Autodesk Fusion 360 part; units mm, degrees
note: some values were not read from the file. Set by a fixed rule: which sketch regions a step uses.
(part 7 of 20)
  spline S36 degree 5 poles (-17.8091, -22.9448) (-17.8092, -22.9448) (-17.8093, -22.945) (-17.8095, -22.9453) (-17.8098, -22.9457) (-17.8103, -22.9463) (-17.8108, -22.9469) (-17.8114, -22.9477) (-17.812, -22.9486) (-17.8127, -22.9496) (-17.8135, -22.9506) (-17.8144, -22.9518) (-17.8153, -22.953) (-17.8162, -22.9543) (-17.8172, -22.9557) (-17.8183, -22.9572) (-17.8195, -22.9588) (-17.8207, -22.9604) (-17.8219, -22.9622) (-17.8232, -22.964) (-17.8246, -22.9659) (-17.826, -22.9679) (-17.8274, -22.9699) (-17.8289, -22.9721) (-17.8305, -22.9743) (-17.8321, -22.9766) (-17.8337, -22.979) (-17.8354, -22.9814) (-17.8372, -22.984) (-17.8389, -22.9866) (-17.8408, -22.9893) (-17.8427, -22.992) (-17.8446, -22.9948) (-17.8465, -22.9978) (-17.8485, -23.0007) (-17.8506, -23.0038) (-17.8527, -23.0069) (-17.8548, -23.0101) (-17.857, -23.0134) (-17.8592, -23.0167) (-17.8614, -23.0201) (-17.8637, -23.0236) (-17.866, -23.0271) (-17.8683, -23.0308) (-17.8707, -23.0344) (-17.8731, -23.0382) (-17.8756, -23.042) (-17.8781, -23.0459) (-17.8806, -23.0499) (-17.8831, -23.0539) (-17.8857, -23.058) (-17.8883, -23.0621) (-17.891, -23.0664) (-17.8937, -23.0706) (-17.8964, -23.075) (-17.8991, -23.0794) (-17.9019, -23.0839) (-17.9047, -23.0884) (-17.9075, -23.093) (-17.9103, -23.0977) (-17.9132, -23.1024) (-17.9161, -23.1072) (-17.9191, -23.1121) (-17.922, -23.117) (-17.925, -23.122) (-17.928, -23.127) (-17.931, -23.1321) (-17.9341, -23.1373) (-17.9372, -23.1425) (-17.9403, -23.1478) (-17.9434, -23.1531) (-17.9466, -23.1585) (-17.9497, -23.164) (-17.9529, -23.1695) (-17.9562, -23.1751) (-17.9594, -23.1807) (-17.9627, -23.1864) (-17.9659, -23.1921) (-17.9692, -23.1979) (-17.9726, -23.2038) (-17.9759, -23.2097) (-17.9793, -23.2157) (-17.9826, -23.2217) (-17.986, -23.2278) (-17.9895, -23.234) (-17.9929, -23.2402) (-17.9963, -23.2464) (-17.9998, -23.2527) (-18.0033, -23.2591) (-18.0068, -23.2655) (-18.0103, -23.272) (-18.0139, -23.2785) (-18.0174, -23.2851) (-18.021, -23.2918) (-18.0246, -23.2984) (-18.0282, -23.3052) (-18.0318, -23.312) (-18.0354, -23.3188) (-18.039, -23.3257) (-18.0427, -23.3327) (-18.0464, -23.3397) (-18.0501, -23.3468) (-18.0538, -23.3539) (-18.0575, -23.361) (-18.0612, -23.3683) (-18.0649, -23.3755) (-18.0687, -23.3828) (-18.0724, -23.3902) (-18.0762, -23.3976) (-18.08, -23.4051) (-18.0838, -23.4126) (-18.0876, -23.4202) (-18.0914, -23.4278) (-18.0952, -23.4355) (-18.0991, -23.4432) (-18.1029, -23.451) (-18.1068, -23.4588) (-18.1106, -23.4666) (-18.1145, -23.4746) (-18.1184, -23.4825) (-18.1223, -23.4905) (-18.1262, -23.4986) (-18.1301, -23.5067) (-18.134, -23.5149) (-18.1379, -23.5231) (-18.1419, -23.5313) (-18.1458, -23.5396) (-18.1498, -23.548) (-18.1537, -23.5564) (-18.1577, -23.5648) (-18.1617, -23.5733) (-18.1657, -23.5818) (-18.1696, -23.5904) (-18.1736, -23.5991) (-18.1776, -23.6077) (-18.1816, -23.6165) (-18.1857, -23.6252) (-18.1897, -23.634) (-18.1937, -23.6429) (-18.1977, -23.6518) (-18.2018, -23.6607) (-18.2058, -23.6697) (-18.2098, -23.6788) (-18.2139, -23.6879) (-18.2179, -23.697) (-18.222, -23.7062) (-18.226, -23.7154) (-18.2301, -23.7247) (-18.2342, -23.734) (-18.2383, -23.7433) (-18.2423, -23.7527) (-18.2464, -23.7622) (-18.2505, -23.7716) (-18.2546, -23.7812) (-18.2587, -23.7907) (-18.2627, -23.8004) (-18.2668, -23.81) (-18.2709, -23.8197) (-18.275, -23.8295) (-18.2791, -23.8393) (-18.2832, -23.8491) (-18.2873, -23.859) (-18.2914, -23.8689) (-18.2955, -23.8788) (-18.2996, -23.8888) (-18.3038, -23.8989) (-18.3079, -23.909) (-18.312, -23.9191) (-18.3161, -23.9292) (-18.3202, -23.9395) (-18.3243, -23.9497) (-18.3284, -23.96) (-18.3325, -23.9703) (-18.3366, -23.9807) (-18.3408, -23.9911) (-18.3449, -24.0016) (-18.349, -24.0121) (-18.3531, -24.0226) (-18.3572, -24.0332) (-18.3613, -24.0438) (-18.3654, -24.0545) (-18.3695, -24.0652) (-18.3736, -24.0759) (-18.3777, -24.0867) (-18.3818, -24.0975) (-18.3859, -24.1084) (-18.39, -24.1193) (-18.3941, -24.1302) (-18.3982, -24.1412) (-18.4023, -24.1522) (-18.4064, -24.1633) (-18.4105, -24.1744) (-18.4146, -24.1855) (-18.4187, -24.1967) (-18.4228, -24.2079) (-18.4269, -24.2191) (-18.4309, -24.2304) (-18.435, -24.2417) (-18.4391, -24.2531) (-18.4431, -24.2645) (-18.4472, -24.276) (-18.4513, -24.2874) (-18.4553, -24.299) (-18.4594, -24.3105) (-18.4634, -24.3221) (-18.4675, -24.3337) (-18.4715, -24.3454) (-18.4756, -24.3571) (-18.4796, -24.3689) (-18.4836, -24.3806) (-18.4877, -24.3925) (-18.4917, -24.4043) (-18.4957, -24.4162) (-18.4997, -24.4281) (-18.5037, -24.4401) (-18.5077, -24.4521) (-18.5117, -24.4642) (-18.5157, -24.4762) (-18.5197, -24.4884) (-18.5237, -24.5005) (-18.5277, -24.5127) (-18.5316, -24.5249) (-18.5356, -24.5372) (-18.5395, -24.5495) (-18.5435, -24.5618) (-18.5475, -24.5742) (-18.5514, -24.5866) (-18.5553, -24.599) (-18.5593, -24.6115) (-18.5632, -24.624) (-18.5671, -24.6365) (-18.571, -24.6491) (-18.5749, -24.6617) (-18.5788, -24.6744) (-18.5827, -24.6871) (-18.5866, -24.6998) (-18.5905, -24.7125) (-18.5943, -24.7253) (-18.5982, -24.7382) (-18.6021, -24.751) (-18.6059, -24.7639) (-18.609, -24.7743) (-18.6113, -24.782) (-18.6128, -24.7872) (-18.6136, -24.7898) knots 0 0 0 0 0 0 0.00416667 0.00833333 0.0125 0.01666667 0.02083333 0.025 0.02916667 0.03333333 0.0375 0.04166667 0.04583333 0.05 0.05416667 0.05833333 0.0625 0.06666667 0.07083333 0.075 0.07916667 0.08333333 0.0875 0.09166667 0.09583333 0.1 0.10416667 0.10833333 0.1125 0.11666667 0.12083333 0.125 0.12916667 0.13333333 0.1375 0.14166667 0.14583333 0.15 0.15416667 0.15833333 0.1625 0.16666667 0.17083333 0.175 0.17916667 0.18333333 0.1875 0.19166667 0.19583333 0.2 0.20416667 0.20833333 0.2125 0.21666667 0.22083333 0.225 0.22916667 0.23333333 0.2375 0.24166667 0.24583333 0.25 0.25416667 0.25833333 0.2625 0.26666667 0.27083333 0.275 0.27916667 0.28333333 0.2875 0.29166667 0.29583333 0.3 0.30416667 0.30833333 0.3125 0.31666667 0.32083333 0.325 0.32916667 0.33333333 0.3375 0.34166667 0.34583333 0.35 0.35416667 0.35833333 0.3625 0.36666667 0.37083333 0.375 0.37916667 0.38333333 0.3875 0.39166667 0.39583333 0.4 0.40416667 0.40833333 0.4125 0.41666667 0.42083333 0.425 0.42916667 0.43333333 0.4375 0.44166667 0.44583333 0.45 0.45416667 0.45833333 0.4625 0.46666667 0.47083333 0.475 0.47916667 0.48333333 0.4875 0.49166667 0.49583333 0.5 0.50416667 0.50833333 0.5125 0.51666667 0.52083333 0.525 0.52916667 0.53333333 0.5375 0.54166667 0.54583333 0.55 0.55416667 0.55833333 0.5625 0.56666667 0.57083333 0.575 0.57916667 0.58333333 0.5875 0.59166667 0.59583333 0.6 0.60416667 0.60833333 0.6125 0.61666667 0.62083333 0.625 0.62916667 0.63333333 0.6375 0.64166667 0.64583333 0.65 0.65416667 0.65833333 0.6625 0.66666667 0.67083333 0.675 0.67916667 0.68333333 0.6875 0.69166667 0.69583333 0.7 0.70416667 0.70833333 0.7125 0.71666667 0.72083333 0.725 0.72916667 0.73333333 0.7375 0.74166667 0.74583333 0.75 0.75416667 0.75833333 0.7625 0.76666667 0.77083333 0.775 0.77916667 0.78333333 0.7875 0.79166667 0.79583333 0.8 0.80416667 0.80833333 0.8125 0.81666667 0.82083333 0.825 0.82916667 0.83333333 0.8375 0.84166667 0.84583333 0.85 0.85416667 0.85833333 0.8625 0.86666667 0.87083333 0.875 0.87916667 0.88333333 0.8875 0.89166667 0.89583333 0.9 0.90416667 0.90833333 0.9125 0.91666667 0.92083333 0.925 0.92916667 0.93333333 0.9375 0.94166667 0.94583333 0.95 0.95416667 0.95833333 0.9625 0.96666667 0.97083333 0.975 0.97916667 0.98333333 0.9875 0.99166667 0.99583333 1 1 1 1 1 1
  spline S37 degree 5 poles (10.0421, -29.3284) (10.0422, -29.3257) (10.0423, -29.3203) (10.0425, -29.3122) (10.0428, -29.3014) (10.0431, -29.288) (10.0434, -29.2745) (10.0437, -29.2612) (10.044, -29.2478) (10.0442, -29.2345) (10.0445, -29.2212) (10.0447, -29.2079) (10.0449, -29.1947) (10.0451, -29.1815) (10.0453, -29.1683) (10.0454, -29.1551) (10.0455, -29.142) (10.0457, -29.129) (10.0458, -29.1159) (10.0458, -29.1029) (10.0459, -29.0899) (10.046, -29.077) (10.046, -29.0641) (10.046, -29.0512) (10.046, -29.0383) (10.046, -29.0255) (10.046, -29.0127) (10.0459, -29) (10.0458, -28.9872) (10.0458, -28.9745) (10.0457, -28.9619) (10.0456, -28.9493) (10.0454, -28.9367) (10.0453, -28.9241) (10.0451, -28.9116) (10.0449, -28.8991) (10.0448, -28.8867) (10.0445, -28.8743) (10.0443, -28.8619) (10.0441, -28.8495) (10.0438, -28.8372) (10.0436, -28.8249) (10.0433, -28.8127) (10.043, -28.8005) (10.0427, -28.7883) (10.0423, -28.7762) (10.042, -28.7641) (10.0416, -28.752) (10.0412, -28.74) (10.0409, -28.728) (10.0405, -28.716) (10.04, -28.7041) (10.0396, -28.6922) (10.0392, -28.6803) (10.0387, -28.6685) (10.0382, -28.6567) (10.0377, -28.645) (10.0372, -28.6333) (10.0367, -28.6216) (10.0362, -28.61) (10.0356, -28.5984) (10.0351, -28.5868) (10.0345, -28.5753) (10.0339, -28.5638) (10.0333, -28.5524) (10.0327, -28.541) (10.0321, -28.5296) (10.0314, -28.5183) (10.0308, -28.507) (10.0301, -28.4957) (10.0294, -28.4845) (10.0287, -28.4733) (10.028, -28.4622) (10.0273, -28.4511) (10.0266, -28.44) (10.0258, -28.429) (10.0251, -28.4181) (10.0243, -28.4071) (10.0235, -28.3962) (10.0227, -28.3854) (10.0219, -28.3745) (10.0211, -28.3638) (10.0203, -28.353) (10.0195, -28.3423) (10.0186, -28.3317) (10.0177, -28.321) (10.0169, -28.3105) (10.016, -28.2999) (10.0151, -28.2894) (10.0142, -28.279) (10.0133, -28.2686) (10.0123, -28.2582) (10.0114, -28.2479) (10.0104, -28.2376) (10.0095, -28.2274) (10.0085, -28.2172) (10.0075, -28.207) (10.0065, -28.1969) (10.0055, -28.1868) (10.0045, -28.1768) (10.0035, -28.1668) (10.0025, -28.1569) (10.0014, -28.147) (10.0004, -28.1372) (9.9993, -28.1274) (9.9983, -28.1176) (9.9972, -28.1079) (9.9961, -28.0982) (9.995, -28.0886) (9.9939, -28.079) (9.9928, -28.0695) (9.9916, -28.06) (9.9905, -28.0506) (9.9894, -28.0412) (9.9882, -28.0318) (9.9871, -28.0225) (9.9859, -28.0133) (9.9847, -28.004) (9.9836, -27.9949) (9.9824, -27.9858) (9.9812, -27.9767) (9.98, -27.9677) (9.9788, -27.9587) (9.9776, -27.9498) (9.9763, -27.9409) (9.9751, -27.9321) (9.9739, -27.9233) (9.9726, -27.9146) (9.9714, -27.9059) (9.9701, -27.8973) (9.9689, -27.8887) (9.9676, -27.8802) (9.9664, -27.8717) (9.9651, -27.8633) (9.9638, -27.8549) (9.9625, -27.8466) (9.9612, -27.8383) (9.9599, -27.8301) (9.9586, -27.8219) (9.9573, -27.8138) (9.956, -27.8057) (9.9547, -27.7977) (9.9534, -27.7898) (9.9521, -27.7819) (9.9508, -27.774) (9.9494, -27.7662) (9.9481, -27.7585) (9.9468, -27.7508) (9.9454, -27.7431) (9.9441, -27.7356) (9.9428, -27.728) (9.9414, -27.7206) (9.9401, -27.7132) (9.9387, -27.7058) (9.9374, -27.6985) (9.936, -27.6912) (9.9347, -27.6841) (9.9333, -27.6769) (9.932, -27.6698) (9.9306, -27.6628) (9.9293, -27.6559) (9.9279, -27.649) (9.9266, -27.6421) (9.9252, -27.6353) (9.9239, -27.6286) (9.9225, -27.622) (9.9212, -27.6154) (9.9199, -27.6088) (9.9185, -27.6023) (9.9172, -27.5959) (9.9158, -27.5896) (9.9145, -27.5833) (9.9132, -27.577) (9.9118, -27.5709) (9.9105, -27.5647) (9.9092, -27.5587) (9.9079, -27.5527) (9.9065, -27.5468) (9.9052, -27.5409) (9.9039, -27.5352) (9.9026, -27.5294) (9.9013, -27.5238) (9.9, -27.5182) (9.8987, -27.5127) (9.8974, -27.5072) (9.8962, -27.5018) (9.8949, -27.4965) (9.8936, -27.4912) (9.8924, -27.4861) (9.8911, -27.481) (9.8899, -27.4759) (9.8887, -27.4709) (9.8874, -27.466) (9.8862, -27.4612) (9.885, -27.4564) (9.8838, -27.4517) (9.8827, -27.4471) (9.8815, -27.4426) (9.8803, -27.4381) (9.8792, -27.4337) (9.878, -27.4294) (9.8769, -27.4252) (9.8758, -27.421) (9.8747, -27.4169) (9.8736, -27.4129) (9.8725, -27.409) (9.8715, -27.4051) (9.8704, -27.4013) (9.8694, -27.3976) (9.8684, -27.394) (9.8674, -27.3905) (9.8664, -27.387) (9.8654, -27.3837) (9.8645, -27.3804) (9.8635, -27.3772) (9.8626, -27.3741) (9.8617, -27.371) (9.8608, -27.3681) (9.86, -27.3652) (9.8591, -27.3625) (9.8583, -27.3598) (9.8575, -27.3572) (9.8568, -27.3547) (9.856, -27.3523) (9.8553, -27.3499) (9.8546, -27.3477) (9.8539, -27.3456) (9.8533, -27.3435) (9.8527, -27.3416) (9.8521, -27.3398) (9.8515, -27.338) (9.851, -27.3364) (9.8505, -27.3348) (9.85, -27.3334) (9.8495, -27.332) (9.8491, -27.3308) (9.8487, -27.3296) (9.8484, -27.3286) (9.8481, -27.3277) (9.8478, -27.3269) (9.8475, -27.3262) (9.8474, -27.3257) (9.8473, -27.3254) (9.8472, -27.3252) (9.8472, -27.3251) knots -1 -1 -1 -1 -1 -1 -0.99583333 -0.99166667 -0.9875 -0.98333333 -0.97916667 -0.975 -0.97083333 -0.96666667 -0.9625 -0.95833333 -0.95416667 -0.95 -0.94583333 -0.94166667 -0.9375 -0.93333333 -0.92916667 -0.925 -0.92083333 -0.91666667 -0.9125 -0.90833333 -0.90416667 -0.9 -0.89583333 -0.89166667 -0.8875 -0.88333333 -0.87916667 -0.875 -0.87083333 -0.86666667 -0.8625 -0.85833333 -0.85416667 -0.85 -0.84583333 -0.84166667 -0.8375 -0.83333333 -0.82916667 -0.825 -0.82083333 -0.81666667 -0.8125 -0.80833333 -0.80416667 -0.8 -0.79583333 -0.79166667 -0.7875 -0.78333333 -0.77916667 -0.775 -0.77083333 -0.76666667 -0.7625 -0.75833333 -0.75416667 -0.75 -0.74583333 -0.74166667 -0.7375 -0.73333333 -0.72916667 -0.725 -0.72083333 -0.71666667 -0.7125 -0.70833333 -0.70416667 -0.7 -0.69583333 -0.69166667 -0.6875 -0.68333333 -0.67916667 -0.675 -0.67083333 -0.66666667 -0.6625 -0.65833333 -0.65416667 -0.65 -0.64583333 -0.64166667 -0.6375 -0.63333333 -0.62916667 -0.625 -0.62083333 -0.61666667 -0.6125 -0.60833333 -0.60416667 -0.6 -0.59583333 -0.59166667 -0.5875 -0.58333333 -0.57916667 -0.575 -0.57083333 -0.56666667 -0.5625 -0.55833333 -0.55416667 -0.55 -0.54583333 -0.54166667 -0.5375 -0.53333333 -0.52916667 -0.525 -0.52083333 -0.51666667 -0.5125 -0.50833333 -0.50416667 -0.5 -0.49583333 -0.49166667 -0.4875 -0.48333333 -0.47916667 -0.475 -0.47083333 -0.46666667 -0.4625 -0.45833333 -0.45416667 -0.45 -0.44583333 -0.44166667 -0.4375 -0.43333333 -0.42916667 -0.425 -0.42083333 -0.41666667 -0.4125 -0.40833333 -0.40416667 -0.4 -0.39583333 -0.39166667 -0.3875 -0.38333333 -0.37916667 -0.375 -0.37083333 -0.36666667 -0.3625 -0.35833333 -0.35416667 -0.35 -0.34583333 -0.34166667 -0.3375 -0.33333333 -0.32916667 -0.325 -0.32083333 -0.31666667 -0.3125 -0.30833333 -0.30416667 -0.3 -0.29583333 -0.29166667 -0.2875 -0.28333333 -0.27916667 -0.275 -0.27083333 -0.26666667 -0.2625 -0.25833333 -0.25416667 -0.25 -0.24583333 -0.24166667 -0.2375 -0.23333333 -0.22916667 -0.225 -0.22083333 -0.21666667 -0.2125 -0.20833333 -0.20416667 -0.2 -0.19583333 -0.19166667 -0.1875 -0.18333333 -0.17916667 -0.175 -0.17083333 -0.16666667 -0.1625 -0.15833333 -0.15416667 -0.15 -0.14583333 -0.14166667 -0.1375 -0.13333333 -0.12916667 -0.125 -0.12083333 -0.11666667 -0.1125 -0.10833333 -0.10416667 -0.1 -0.09583333 -0.09166667 -0.0875 -0.08333333 -0.07916667 -0.075 -0.07083333 -0.06666667 -0.0625 -0.05833333 -0.05416667 -0.05 -0.04583333 -0.04166667 -0.0375 -0.03333333 -0.02916667 -0.025 -0.02083333 -0.01666667 -0.0125 -0.00833333 -0.00416667 0 0 0 0 0 0
  arc A39 (-15.9204, -26.5997) -> (-15.0758, -27.0873) centre (0, 0) ccw
  arc A40 (22.7115, 17.6281) -> (21.9649, 18.5501) centre (0, 0) ccw
  arc A41 (12.5209, -25.8803) -> (13.578, -25.3417) centre (0, 0) ccw
  line L88 (-25.3417, -13.578) -> (-25.6012, -13.7171)
  line L89 (-28.587, -5.1345) -> (-28.5878, -5.1346)
  spline S38 degree 5 poles (28.7753, -3.9508) (28.7754, -3.9508) (28.7756, -3.9508) (28.7759, -3.9509) (28.7764, -3.9509) (28.7772, -3.951) (28.778, -3.9511) (28.779, -3.9512) (28.7801, -3.9514) (28.7813, -3.9515) (28.7826, -3.9517) (28.784, -3.9518) (28.7855, -3.952) (28.7871, -3.9522) (28.7889, -3.9523) (28.7907, -3.9525) (28.7926, -3.9527) (28.7946, -3.9529) (28.7968, -3.9531) (28.799, -3.9534) (28.8013, -3.9536) (28.8037, -3.9538) (28.8063, -3.954) (28.8089, -3.9543) (28.8116, -3.9545) (28.8144, -3.9547) (28.8172, -3.955) (28.8202, -3.9552) (28.8233, -3.9555) (28.8264, -3.9557) (28.8297, -3.9559) (28.833, -3.9562) (28.8364, -3.9564) (28.8399, -3.9567) (28.8435, -3.9569) (28.8472, -3.9572) (28.8509, -3.9574) (28.8547, -3.9577) (28.8586, -3.9579) (28.8626, -3.9581) (28.8667, -3.9584) (28.8709, -3.9586) (28.8751, -3.9588) (28.8794, -3.959) (28.8838, -3.9593) (28.8882, -3.9595) (28.8928, -3.9597) (28.8974, -3.9599) (28.9021, -3.9601) (28.9068, -3.9603) (28.9117, -3.9605) (28.9166, -3.9607) (28.9215, -3.9609) (28.9266, -3.961) (28.9317, -3.9612) (28.9369, -3.9614) (28.9422, -3.9615) (28.9475, -3.9617) (28.9529, -3.9618) (28.9584, -3.962) (28.9639, -3.9621) (28.9695, -3.9622) (28.9752, -3.9623) (28.9809, -3.9624) (28.9867, -3.9625) (28.9926, -3.9626) (28.9985, -3.9627) (29.0045, -3.9627) (29.0106, -3.9628) (29.0167, -3.9629) (29.0229, -3.9629) (29.0291, -3.9629) (29.0355, -3.9629) (29.0418, -3.963) (29.0483, -3.963) (29.0548, -3.9629) (29.0613, -3.9629) (29.068, -3.9629) (29.0746, -3.9628) (29.0814, -3.9628) (29.0882, -3.9627) (29.095, -3.9626) (29.1019, -3.9626) (29.1089, -3.9625) (29.1159, -3.9623) (29.123, -3.9622) (29.1302, -3.9621) (29.1374, -3.9619) (29.1446, -3.9618) (29.1519, -3.9616) (29.1593, -3.9614) (29.1667, -3.9612) (29.1742, -3.961) (29.1817, -3.9607) (29.1893, -3.9605) (29.197, -3.9603) (29.2047, -3.96) (29.2124, -3.9597) (29.2202, -3.9594) (29.2281, -3.9591) (29.236, -3.9588) (29.2439, -3.9584) (29.2519, -3.9581) (29.26, -3.9577) (29.2681, -3.9573) (29.2763, -3.9569) (29.2845, -3.9565) (29.2927, -3.9561) (29.301, -3.9556) (29.3094, -3.9552) (29.3178, -3.9547) (29.3263, -3.9542) (29.3348, -3.9537) (29.3433, -3.9532) (29.3519, -3.9526) (29.3606, -3.9521) (29.3693, -3.9515) (29.378, -3.9509) (29.3868, -3.9503) (29.3957, -3.9497) (29.4045, -3.9491) (29.4135, -3.9484) (29.4225, -3.9478) (29.4315, -3.9471) (29.4406, -3.9464) (29.4497, -3.9457) (29.4588, -3.9449) (29.468, -3.9442) (29.4773, -3.9434) (29.4866, -3.9426) (29.4959, -3.9418) (29.5053, -3.941) (29.5147, -3.9402) (29.5242, -3.9393) (29.5337, -3.9384) (29.5433, -3.9375) (29.5529, -3.9366) (29.5625, -3.9357) (29.5722, -3.9348) (29.5819, -3.9338) (29.5917, -3.9328) (29.6015, -3.9318) (29.6113, -3.9308) (29.6212, -3.9297) (29.6312, -3.9287) (29.6411, -3.9276) (29.6512, -3.9265) (29.6612, -3.9254) (29.6713, -3.9243) (29.6814, -3.9231) (29.6916, -3.922) (29.7018, -3.9208) (29.7121, -3.9196) (29.7224, -3.9183) (29.7327, -3.9171) (29.7431, -3.9158) (29.7535, -3.9145) (29.764, -3.9132) (29.7744, -3.9119) (29.785, -3.9106) (29.7955, -3.9092) (29.8061, -3.9078) (29.8168, -3.9064) (29.8274, -3.905) (29.8382, -3.9035) (29.8489, -3.9021) (29.8597, -3.9006) (29.8705, -3.8991) (29.8814, -3.8976) (29.8923, -3.896) (29.9032, -3.8945) (29.9142, -3.8929) (29.9252, -3.8913) (29.9362, -3.8896) (29.9473, -3.888) (29.9584, -3.8863) (29.9696, -3.8846) (29.9807, -3.8829) (29.992, -3.8812) (30.0032, -3.8795) (30.0145, -3.8777) (30.0258, -3.8759) (30.0372, -3.8741) (30.0486, -3.8722) (30.06, -3.8704) (30.0714, -3.8685) (30.0829, -3.8666) (30.0944, -3.8647) (30.106, -3.8628) (30.1176, -3.8608) (30.1292, -3.8588) (30.1409, -3.8568) (30.1525, -3.8548) (30.1643, -3.8527) (30.176, -3.8507) (30.1878, -3.8486) (30.1996, -3.8464) (30.2115, -3.8443) (30.2233, -3.8422) (30.2353, -3.84) (30.2472, -3.8378) (30.2592, -3.8356) (30.2712, -3.8333) (30.2832, -3.831) (30.2953, -3.8288) (30.3074, -3.8264) (30.3195, -3.8241) (30.3317, -3.8217) (30.3439, -3.8194) (30.3561, -3.817) (30.3683, -3.8145) (30.3806, -3.8121) (30.3929, -3.8096) (30.4053, -3.8071) (30.4176, -3.8046) (30.43, -3.8021) (30.4424, -3.7995) (30.4549, -3.797) (30.4674, -3.7943) (30.4799, -3.7917) (30.4924, -3.7891) (30.505, -3.7864) (30.5176, -3.7837) (30.5302, -3.781) (30.5429, -3.7782) (30.5556, -3.7755) (30.5683, -3.7727) (30.581, -3.7699) (30.5938, -3.767) (30.6066, -3.7642) (30.6194, -3.7613) (30.6323, -3.7584) (30.6451, -3.7555) (30.658, -3.7525) (30.671, -3.7496) (30.6839, -3.7466) (30.6969, -3.7435) (30.7099, -3.7405) (30.723, -3.7374) (30.736, -3.7343) (30.7491, -3.7312) (30.7596, -3.7287) (30.7675, -3.7268) (30.7728, -3.7256) (30.7754, -3.7249) knots 0 0 0 0 0 0 0.00416667 0.00833333 0.0125 0.01666667 0.02083333 0.025 0.02916667 0.03333333 0.0375 0.04166667 0.04583333 0.05 0.05416667 0.05833333 0.0625 0.06666667 0.07083333 0.075 0.07916667 0.08333333 0.0875 0.09166667 0.09583333 0.1 0.10416667 0.10833333 0.1125 0.11666667 0.12083333 0.125 0.12916667 0.13333333 0.1375 0.14166667 0.14583333 0.15 0.15416667 0.15833333 0.1625 0.16666667 0.17083333 0.175 0.17916667 0.18333333 0.1875 0.19166667 0.19583333 0.2 0.20416667 0.20833333 0.2125 0.21666667 0.22083333 0.225 0.22916667 0.23333333 0.2375 0.24166667 0.24583333 0.25 0.25416667 0.25833333 0.2625 0.26666667 0.27083333 0.275 0.27916667 0.28333333 0.2875 0.29166667 0.29583333 0.3 0.30416667 0.30833333 0.3125 0.31666667 0.32083333 0.325 0.32916667 0.33333333 0.3375 0.34166667 0.34583333 0.35 0.35416667 0.35833333 0.3625 0.36666667 0.37083333 0.375 0.37916667 0.38333333 0.3875 0.39166667 0.39583333 0.4 0.40416667 0.40833333 0.4125 0.41666667 0.42083333 0.425 0.42916667 0.43333333 0.4375 0.44166667 0.44583333 0.45 0.45416667 0.45833333 0.4625 0.46666667 0.47083333 0.475 0.47916667 0.48333333 0.4875 0.49166667 0.49583333 0.5 0.50416667 0.50833333 0.5125 0.51666667 0.52083333 0.525 0.52916667 0.53333333 0.5375 0.54166667 0.54583333 0.55 0.55416667 0.55833333 0.5625 0.56666667 0.57083333 0.575 0.57916667 0.58333333 0.5875 0.59166667 0.59583333 0.6 0.60416667 0.60833333 0.6125 0.61666667 0.62083333 0.625 0.62916667 0.63333333 0.6375 0.64166667 0.64583333 0.65 0.65416667 0.65833333 0.6625 0.66666667 0.67083333 0.675 0.67916667 0.68333333 0.6875 0.69166667 0.69583333 0.7 0.70416667 0.70833333 0.7125 0.71666667 0.72083333 0.725 0.72916667 0.73333333 0.7375 0.74166667 0.74583333 0.75 0.75416667 0.75833333 0.7625 0.76666667 0.77083333 0.775 0.77916667 0.78333333 0.7875 0.79166667 0.79583333 0.8 0.80416667 0.80833333 0.8125 0.81666667 0.82083333 0.825 0.82916667 0.83333333 0.8375 0.84166667 0.84583333 0.85 0.85416667 0.85833333 0.8625 0.86666667 0.87083333 0.875 0.87916667 0.88333333 0.8875 0.89166667 0.89583333 0.9 0.90416667 0.90833333 0.9125 0.91666667 0.92083333 0.925 0.92916667 0.93333333 0.9375 0.94166667 0.94583333 0.95 0.95416667 0.95833333 0.9625 0.96666667 0.97083333 0.975 0.97916667 0.98333333 0.9875 0.99166667 0.99583333 1 1 1 1 1 1
  line L90 (-26.1453, -12.6491) -> (-25.8803, -12.5209)
  line L91 (-23.7836, -16.1526) -> (-24.0271, -16.318)
  line L92 (-24.6799, -15.3128) -> (-24.4297, -15.1575)
  spline S39 degree 5 poles (29.6298, -9.1146) (29.6276, -9.1129) (29.6234, -9.1096) (29.6169, -9.1047) (29.6084, -9.0981) (29.5977, -9.09) (29.587, -9.0818) (29.5763, -9.0737) (29.5657, -9.0657) (29.555, -9.0576) (29.5444, -9.0496) (29.5338, -9.0416) (29.5232, -9.0337) (29.5127, -9.0258) (29.5021, -9.0179) (29.4915, -9.0101) (29.481, -9.0022) (29.4705, -8.9945) (29.46, -8.9867) (29.4495, -8.979) (29.4391, -8.9713) (29.4286, -8.9637) (29.4182, -8.956) (29.4078, -8.9485) (29.3974, -8.9409) (29.387, -8.9334) (29.3766, -8.9259) (29.3663, -8.9184) (29.356, -8.911) (29.3457, -8.9036) (29.3354, -8.8963) (29.3251, -8.8889) (29.3148, -8.8816) (29.3046, -8.8744) (29.2944, -8.8671) (29.2842, -8.86) (29.274, -8.8528) (29.2638, -8.8457) (29.2537, -8.8386) (29.2435, -8.8315) (29.2334, -8.8245) (29.2233, -8.8175) (29.2132, -8.8105) (29.2032, -8.8036) (29.1932, -8.7967) (29.1831, -8.7898) (29.1731, -8.783) (29.1632, -8.7762) (29.1532, -8.7694) (29.1433, -8.7626) (29.1334, -8.7559) (29.1235, -8.7493) (29.1136, -8.7426) (29.1037, -8.736) (29.0939, -8.7295) (29.0841, -8.7229) (29.0743, -8.7164) (29.0646, -8.7099) (29.0548, -8.7035) (29.0451, -8.6971) (29.0354, -8.6907) (29.0257, -8.6844) (29.016, -8.6781) (29.0064, -8.6718) (28.9968, -8.6656) (28.9872, -8.6593) (28.9776, -8.6532) (28.9681, -8.647) (28.9586, -8.6409) (28.9491, -8.6348) (28.9396, -8.6288) (28.9302, -8.6228) (28.9207, -8.6168) (28.9113, -8.6109) (28.902, -8.605) (28.8926, -8.5991) (28.8833, -8.5932) (28.874, -8.5874) (28.8647, -8.5817) (28.8555, -8.5759) (28.8462, -8.5702) (28.837, -8.5645) (28.8279, -8.5589) (28.8187, -8.5533) (28.8096, -8.5477) (28.8005, -8.5422) (28.7914, -8.5367) (28.7824, -8.5312) (28.7734, -8.5257) (28.7644, -8.5203) (28.7554, -8.515) (28.7465, -8.5096) (28.7376, -8.5043) (28.7287, -8.499) (28.7199, -8.4938) (28.711, -8.4886) (28.7022, -8.4834) (28.6935, -8.4783) (28.6847, -8.4732) (28.676, -8.4681) (28.6674, -8.463) (28.6587, -8.458) (28.6501, -8.4531) (28.6415, -8.4481) (28.633, -8.4432) (28.6244, -8.4384) (28.616, -8.4335) (28.6075, -8.4287) (28.5991, -8.4239) (28.5907, -8.4192) (28.5823, -8.4145) (28.574, -8.4098) (28.5657, -8.4052) (28.5574, -8.4006) (28.5491, -8.396) (28.5409, -8.3915) (28.5328, -8.387) (28.5246, -8.3825) (28.5165, -8.3781) (28.5085, -8.3737) (28.5004, -8.3693) (28.4924, -8.365) (28.4845, -8.3607) (28.4765, -8.3565) (28.4686, -8.3522) (28.4608, -8.348) (28.4529, -8.3439) (28.4452, -8.3398) (28.4374, -8.3357) (28.4297, -8.3316) (28.422, -8.3276) (28.4144, -8.3236) (28.4068, -8.3196) (28.3992, -8.3157) (28.3917, -8.3118) (28.3842, -8.308) (28.3767, -8.3042) (28.3693, -8.3004) (28.3619, -8.2966) (28.3546, -8.2929) (28.3473, -8.2892) (28.3401, -8.2856) (28.3329, -8.282) (28.3257, -8.2784) (28.3186, -8.2748) (28.3115, -8.2713) (28.3044, -8.2678) (28.2974, -8.2644) (28.2905, -8.261) (28.2835, -8.2576) (28.2767, -8.2543) (28.2698, -8.251) (28.263, -8.2477) (28.2563, -8.2445) (28.2496, -8.2412) (28.2429, -8.2381) (28.2363, -8.2349) (28.2298, -8.2318) (28.2233, -8.2288) (28.2168, -8.2257) (28.2104, -8.2227) (28.204, -8.2198) (28.1977, -8.2169) (28.1914, -8.214) (28.1851, -8.2111) (28.179, -8.2083) (28.1728, -8.2055) (28.1667, -8.2027) (28.1607, -8.2) (28.1547, -8.1973) (28.1488, -8.1947) (28.1429, -8.192) (28.1371, -8.1895) (28.1313, -8.1869) (28.1256, -8.1844) (28.1199, -8.1819) (28.1143, -8.1795) (28.1087, -8.177) (28.1032, -8.1747) (28.0978, -8.1723) (28.0924, -8.17) (28.087, -8.1677) (28.0818, -8.1655) (28.0765, -8.1633) (28.0714, -8.1611) (28.0663, -8.159) (28.0612, -8.1569) (28.0562, -8.1548) (28.0513, -8.1528) (28.0464, -8.1508) (28.0416, -8.1488) (28.0369, -8.1469) (28.0322, -8.145) (28.0276, -8.1432) (28.023, -8.1413) (28.0185, -8.1395) (28.0141, -8.1378) (28.0097, -8.1361) (28.0054, -8.1344) (28.0012, -8.1327) (27.997, -8.1311) (27.9929, -8.1295) (27.9889, -8.128) (27.9849, -8.1265) (27.9811, -8.125) (27.9772, -8.1236) (27.9735, -8.1222) (27.9698, -8.1208) (27.9662, -8.1194) (27.9627, -8.1181) (27.9593, -8.1169) (27.9559, -8.1156) (27.9526, -8.1144) (27.9494, -8.1133) (27.9462, -8.1121) (27.9432, -8.1111) (27.9402, -8.11) (27.9373, -8.109) (27.9345, -8.108) (27.9318, -8.107) (27.9291, -8.1061) (27.9265, -8.1052) (27.9241, -8.1044) (27.9217, -8.1036) (27.9194, -8.1028) (27.9172, -8.102) (27.915, -8.1013) (27.913, -8.1007) (27.9111, -8.1) (27.9092, -8.0994) (27.9075, -8.0988) (27.9058, -8.0983) (27.9043, -8.0978) (27.9028, -8.0973) (27.9015, -8.0969) (27.9002, -8.0965) (27.8991, -8.0962) (27.898, -8.0958) (27.8971, -8.0956) (27.8963, -8.0953) (27.8956, -8.0951) (27.8951, -8.0949) (27.8948, -8.0948) (27.8946, -8.0948) (27.8945, -8.0948) knots -1 -1 -1 -1 -1 -1 -0.99583333 -0.99166667 -0.9875 -0.98333333 -0.97916667 -0.975 -0.97083333 -0.96666667 -0.9625 -0.95833333 -0.95416667 -0.95 -0.94583333 -0.94166667 -0.9375 -0.93333333 -0.92916667 -0.925 -0.92083333 -0.91666667 -0.9125 -0.90833333 -0.90416667 -0.9 -0.89583333 -0.89166667 -0.8875 -0.88333333 -0.87916667 -0.875 -0.87083333 -0.86666667 -0.8625 -0.85833333 -0.85416667 -0.85 -0.84583333 -0.84166667 -0.8375 -0.83333333 -0.82916667 -0.825 -0.82083333 -0.81666667 -0.8125 -0.80833333 -0.80416667 -0.8 -0.79583333 -0.79166667 -0.7875 -0.78333333 -0.77916667 -0.775 -0.77083333 -0.76666667 -0.7625 -0.75833333 -0.75416667 -0.75 -0.74583333 -0.74166667 -0.7375 -0.73333333 -0.72916667 -0.725 -0.72083333 -0.71666667 -0.7125 -0.70833333 -0.70416667 -0.7 -0.69583333 -0.69166667 -0.6875 -0.68333333 -0.67916667 -0.675 -0.67083333 -0.66666667 -0.6625 -0.65833333 -0.65416667 -0.65 -0.64583333 -0.64166667 -0.6375 -0.63333333 -0.62916667 -0.625 -0.62083333 -0.61666667 -0.6125 -0.60833333 -0.60416667 -0.6 -0.59583333 -0.59166667 -0.5875 -0.58333333 -0.57916667 -0.575 -0.57083333 -0.56666667 -0.5625 -0.55833333 -0.55416667 -0.55 -0.54583333 -0.54166667 -0.5375 -0.53333333 -0.52916667 -0.525 -0.52083333 -0.51666667 -0.5125 -0.50833333 -0.50416667 -0.5 -0.49583333 -0.49166667 -0.4875 -0.48333333 -0.47916667 -0.475 -0.47083333 -0.46666667 -0.4625 -0.45833333 -0.45416667 -0.45 -0.44583333 -0.44166667 -0.4375 -0.43333333 -0.42916667 -0.425 -0.42083333 -0.41666667 -0.4125 -0.40833333 -0.40416667 -0.4 -0.39583333 -0.39166667 -0.3875 -0.38333333 -0.37916667 -0.375 -0.37083333 -0.36666667 -0.3625 -0.35833333 -0.35416667 -0.35 -0.34583333 -0.34166667 -0.3375 -0.33333333 -0.32916667 -0.325 -0.32083333 -0.31666667 -0.3125 -0.30833333 -0.30416667 -0.3 -0.29583333 -0.29166667 -0.2875 -0.28333333 -0.27916667 -0.275 -0.27083333 -0.26666667 -0.2625 -0.25833333 -0.25416667 -0.25 -0.24583333 -0.24166667 -0.2375 -0.23333333 -0.22916667 -0.225 -0.22083333 -0.21666667 -0.2125 -0.20833333 -0.20416667 -0.2 -0.19583333 -0.19166667 -0.1875 -0.18333333 -0.17916667 -0.175 -0.17083333 -0.16666667 -0.1625 -0.15833333 -0.15416667 -0.15 -0.14583333 -0.14166667 -0.1375 -0.13333333 -0.12916667 -0.125 -0.12083333 -0.11666667 -0.1125 -0.10833333 -0.10416667 -0.1 -0.09583333 -0.09166667 -0.0875 -0.08333333 -0.07916667 -0.075 -0.07083333 -0.06666667 -0.0625 -0.05833333 -0.05416667 -0.05 -0.04583333 -0.04166667 -0.0375 -0.03333333 -0.02916667 -0.025 -0.02083333 -0.01666667 -0.0125 -0.00833333 -0.00416667 0 0 0 0 0 0
  line L93 (-25.6012, -13.7171) -> (-25.6019, -13.7175)
  arc A42 (26.6221, -10.8547) -> (27.0473, -9.7471) centre (0, 0) ccw
  spline S40 degree 5 poles (-30.7754, -3.7249) (-30.7728, -3.7256) (-30.7675, -3.7268) (-30.7596, -3.7287) (-30.7491, -3.7312) (-30.736, -3.7343) (-30.723, -3.7374) (-30.7099, -3.7405) (-30.6969, -3.7435) (-30.6839, -3.7466) (-30.671, -3.7496) (-30.658, -3.7525) (-30.6451, -3.7555) (-30.6323, -3.7584) (-30.6194, -3.7613) (-30.6066, -3.7642) (-30.5938, -3.767) (-30.581, -3.7699) (-30.5683, -3.7727) (-30.5556, -3.7755) (-30.5429, -3.7782) (-30.5302, -3.781) (-30.5176, -3.7837) (-30.505, -3.7864) (-30.4924, -3.7891) (-30.4799, -3.7917) (-30.4674, -3.7943) (-30.4549, -3.797) (-30.4424, -3.7995) (-30.43, -3.8021) (-30.4176, -3.8046) (-30.4053, -3.8071) (-30.3929, -3.8096) (-30.3806, -3.8121) (-30.3683, -3.8145) (-30.3561, -3.817) (-30.3439, -3.8194) (-30.3317, -3.8217) (-30.3195, -3.8241) (-30.3074, -3.8264) (-30.2953, -3.8288) (-30.2832, -3.831) (-30.2712, -3.8333) (-30.2592, -3.8356) (-30.2472, -3.8378) (-30.2353, -3.84) (-30.2233, -3.8422) (-30.2115, -3.8443) (-30.1996, -3.8464) (-30.1878, -3.8486) (-30.176, -3.8507) (-30.1643, -3.8527) (-30.1525, -3.8548) (-30.1409, -3.8568) (-30.1292, -3.8588) (-30.1176, -3.8608) (-30.106, -3.8628) (-30.0944, -3.8647) (-30.0829, -3.8666) (-30.0714, -3.8685) (-30.06, -3.8704) (-30.0486, -3.8722) (-30.0372, -3.8741) (-30.0258, -3.8759) (-30.0145, -3.8777) (-30.0032, -3.8795) (-29.992, -3.8812) (-29.9807, -3.8829) (-29.9696, -3.8846) (-29.9584, -3.8863) (-29.9473, -3.888) (-29.9362, -3.8896) (-29.9252, -3.8913) (-29.9142, -3.8929) (-29.9032, -3.8945) (-29.8923, -3.896) (-29.8814, -3.8976) (-29.8705, -3.8991) (-29.8597, -3.9006) (-29.8489, -3.9021) (-29.8382, -3.9035) (-29.8274, -3.905) (-29.8168, -3.9064) (-29.8061, -3.9078) (-29.7955, -3.9092) (-29.785, -3.9106) (-29.7744, -3.9119) (-29.764, -3.9132) (-29.7535, -3.9145) (-29.7431, -3.9158) (-29.7327, -3.9171) (-29.7224, -3.9183) (-29.7121, -3.9196) (-29.7018, -3.9208) (-29.6916, -3.922) (-29.6814, -3.9231) (-29.6713, -3.9243) (-29.6612, -3.9254) (-29.6512, -3.9265) (-29.6411, -3.9276) (-29.6312, -3.9287) (-29.6212, -3.9297) (-29.6113, -3.9308) (-29.6015, -3.9318) (-29.5917, -3.9328) (-29.5819, -3.9338) (-29.5722, -3.9348) (-29.5625, -3.9357) (-29.5529, -3.9366) (-29.5433, -3.9375) (-29.5337, -3.9384) (-29.5242, -3.9393) (-29.5147, -3.9402) (-29.5053, -3.941) (-29.4959, -3.9418) (-29.4866, -3.9426) (-29.4773, -3.9434) (-29.468, -3.9442) (-29.4588, -3.9449) (-29.4497, -3.9457) (-29.4406, -3.9464) (-29.4315, -3.9471) (-29.4225, -3.9478) (-29.4135, -3.9484) (-29.4045, -3.9491) (-29.3957, -3.9497) (-29.3868, -3.9503) (-29.378, -3.9509) (-29.3693, -3.9515) (-29.3606, -3.9521) (-29.3519, -3.9526) (-29.3433, -3.9532) (-29.3348, -3.9537) (-29.3263, -3.9542) (-29.3178, -3.9547) (-29.3094, -3.9552) (-29.301, -3.9556) (-29.2927, -3.9561) (-29.2845, -3.9565) (-29.2763, -3.9569) (-29.2681, -3.9573) (-29.26, -3.9577) (-29.2519, -3.9581) (-29.2439, -3.9584) (-29.236, -3.9588) (-29.2281, -3.9591) (-29.2202, -3.9594) (-29.2124, -3.9597) (-29.2047, -3.96) (-29.197, -3.9603) (-29.1893, -3.9605) (-29.1817, -3.9607) (-29.1742, -3.961) (-29.1667, -3.9612) (-29.1593, -3.9614) (-29.1519, -3.9616) (-29.1446, -3.9618) (-29.1374, -3.9619) (-29.1302, -3.9621) (-29.123, -3.9622) (-29.1159, -3.9623) (-29.1089, -3.9625) (-29.1019, -3.9626) (-29.095, -3.9626) (-29.0882, -3.9627) (-29.0814, -3.9628) (-29.0746, -3.9628) (-29.068, -3.9629) (-29.0613, -3.9629) (-29.0548, -3.9629) (-29.0483, -3.963) (-29.0418, -3.963) (-29.0355, -3.9629) (-29.0291, -3.9629) (-29.0229, -3.9629) (-29.0167, -3.9629) (-29.0106, -3.9628) (-29.0045, -3.9627) (-28.9985, -3.9627) (-28.9926, -3.9626) (-28.9867, -3.9625) (-28.9809, -3.9624) (-28.9752, -3.9623) (-28.9695, -3.9622) (-28.9639, -3.9621) (-28.9584, -3.962) (-28.9529, -3.9618) (-28.9475, -3.9617) (-28.9422, -3.9615) (-28.9369, -3.9614) (-28.9317, -3.9612) (-28.9266, -3.961) (-28.9215, -3.9609) (-28.9166, -3.9607) (-28.9117, -3.9605) (-28.9068, -3.9603) (-28.9021, -3.9601) (-28.8974, -3.9599) (-28.8928, -3.9597) (-28.8882, -3.9595) (-28.8838, -3.9593) (-28.8794, -3.959) (-28.8751, -3.9588) (-28.8709, -3.9586) (-28.8667, -3.9584) (-28.8626, -3.9581) (-28.8586, -3.9579) (-28.8547, -3.9577) (-28.8509, -3.9574) (-28.8472, -3.9572) (-28.8435, -3.9569) (-28.8399, -3.9567) (-28.8364, -3.9564) (-28.833, -3.9562) (-28.8297, -3.9559) (-28.8264, -3.9557) (-28.8233, -3.9555) (-28.8202, -3.9552) (-28.8172, -3.955) (-28.8144, -3.9547) (-28.8116, -3.9545) (-28.8089, -3.9543) (-28.8063, -3.954) (-28.8037, -3.9538) (-28.8013, -3.9536) (-28.799, -3.9534) (-28.7968, -3.9531) (-28.7946, -3.9529) (-28.7926, -3.9527) (-28.7907, -3.9525) (-28.7889, -3.9523) (-28.7871, -3.9522) (-28.7855, -3.952) (-28.784, -3.9518) (-28.7826, -3.9517) (-28.7813, -3.9515) (-28.7801, -3.9514) (-28.779, -3.9512) (-28.778, -3.9511) (-28.7772, -3.951) (-28.7764, -3.9509) (-28.7759, -3.9509) (-28.7756, -3.9508) (-28.7754, -3.9508) (-28.7753, -3.9508) knots -1 -1 -1 -1 -1 -1 -0.99583333 -0.99166667 -0.9875 -0.98333333 -0.97916667 -0.975 -0.97083333 -0.96666667 -0.9625 -0.95833333 -0.95416667 -0.95 -0.94583333 -0.94166667 -0.9375 -0.93333333 -0.92916667 -0.925 -0.92083333 -0.91666667 -0.9125 -0.90833333 -0.90416667 -0.9 -0.89583333 -0.89166667 -0.8875 -0.88333333 -0.87916667 -0.875 -0.87083333 -0.86666667 -0.8625 -0.85833333 -0.85416667 -0.85 -0.84583333 -0.84166667 -0.8375 -0.83333333 -0.82916667 -0.825 -0.82083333 -0.81666667 -0.8125 -0.80833333 -0.80416667 -0.8 -0.79583333 -0.79166667 -0.7875 -0.78333333 -0.77916667 -0.775 -0.77083333 -0.76666667 -0.7625 -0.75833333 -0.75416667 -0.75 -0.74583333 -0.74166667 -0.7375 -0.73333333 -0.72916667 -0.725 -0.72083333 -0.71666667 -0.7125 -0.70833333 -0.70416667 -0.7 -0.69583333 -0.69166667 -0.6875 -0.68333333 -0.67916667 -0.675 -0.67083333 -0.66666667 -0.6625 -0.65833333 -0.65416667 -0.65 -0.64583333 -0.64166667 -0.6375 -0.63333333 -0.62916667 -0.625 -0.62083333 -0.61666667 -0.6125 -0.60833333 -0.60416667 -0.6 -0.59583333 -0.59166667 -0.5875 -0.58333333 -0.57916667 -0.575 -0.57083333 -0.56666667 -0.5625 -0.55833333 -0.55416667 -0.55 -0.54583333 -0.54166667 -0.5375 -0.53333333 -0.52916667 -0.525 -0.52083333 -0.51666667 -0.5125 -0.50833333 -0.50416667 -0.5 -0.49583333 -0.49166667 -0.4875 -0.48333333 -0.47916667 -0.475 -0.47083333 -0.46666667 -0.4625 -0.45833333 -0.45416667 -0.45 -0.44583333 -0.44166667 -0.4375 -0.43333333 -0.42916667 -0.425 -0.42083333 -0.41666667 -0.4125 -0.40833333 -0.40416667 -0.4 -0.39583333 -0.39166667 -0.3875 -0.38333333 -0.37916667 -0.375 -0.37083333 -0.36666667 -0.3625 -0.35833333 -0.35416667 -0.35 -0.34583333 -0.34166667 -0.3375 -0.33333333 -0.32916667 -0.325 -0.32083333 -0.31666667 -0.3125 -0.30833333 -0.30416667 -0.3 -0.29583333 -0.29166667 -0.2875 -0.28333333 -0.27916667 -0.275 -0.27083333 -0.26666667 -0.2625 -0.25833333 -0.25416667 -0.25 -0.24583333 -0.24166667 -0.2375 -0.23333333 -0.22916667 -0.225 -0.22083333 -0.21666667 -0.2125 -0.20833333 -0.20416667 -0.2 -0.19583333 -0.19166667 -0.1875 -0.18333333 -0.17916667 -0.175 -0.17083333 -0.16666667 -0.1625 -0.15833333 -0.15416667 -0.15 -0.14583333 -0.14166667 -0.1375 -0.13333333 -0.12916667 -0.125 -0.12083333 -0.11666667 -0.1125 -0.10833333 -0.10416667 -0.1 -0.09583333 -0.09166667 -0.0875 -0.08333333 -0.07916667 -0.075 -0.07083333 -0.06666667 -0.0625 -0.05833333 -0.05416667 -0.05 -0.04583333 -0.04166667 -0.0375 -0.03333333 -0.02916667 -0.025 -0.02083333 -0.01666667 -0.0125 -0.00833333 -0.00416667 0 0 0 0 0 0
  line L94 (-26.1461, -12.6495) -> (-26.1453, -12.6491)
  spline S41 degree 5 poles (28.2047, -6.937) (28.2048, -6.937) (28.205, -6.937) (28.2053, -6.9371) (28.2058, -6.9372) (28.2065, -6.9374) (28.2074, -6.9376) (28.2083, -6.9378) (28.2094, -6.9381) (28.2106, -6.9383) (28.2118, -6.9386) (28.2132, -6.9389) (28.2147, -6.9392) (28.2163, -6.9396) (28.218, -6.9399) (28.2198, -6.9403) (28.2217, -6.9407) (28.2237, -6.9411) (28.2258, -6.9416) (28.228, -6.942) (28.2303, -6.9425) (28.2327, -6.9429) (28.2351, -6.9434) (28.2377, -6.9439) (28.2404, -6.9445) (28.2431, -6.945) (28.246, -6.9455) (28.2489, -6.9461) (28.2519, -6.9466) (28.255, -6.9472) (28.2582, -6.9478) (28.2615, -6.9484) (28.2649, -6.949) (28.2683, -6.9496) (28.2719, -6.9502) (28.2755, -6.9508) (28.2792, -6.9515) (28.283, -6.9521) (28.2868, -6.9528) (28.2908, -6.9534) (28.2948, -6.9541) (28.2989, -6.9547) (28.3031, -6.9554) (28.3074, -6.9561) (28.3117, -6.9568) (28.3161, -6.9574) (28.3206, -6.9581) (28.3252, -6.9588) (28.3298, -6.9595) (28.3345, -6.9602) (28.3393, -6.9609) (28.3442, -6.9616) (28.3491, -6.9623) (28.3541, -6.963) (28.3592, -6.9637) (28.3643, -6.9644) (28.3695, -6.9651) (28.3748, -6.9658) (28.3802, -6.9665) (28.3856, -6.9672) (28.3911, -6.9679) (28.3966, -6.9686) (28.4023, -6.9693) (28.408, -6.97) (28.4137, -6.9707) (28.4196, -6.9714) (28.4255, -6.9721) (28.4314, -6.9728) (28.4374, -6.9735) (28.4435, -6.9742) (28.4497, -6.9749) (28.4559, -6.9756) (28.4622, -6.9763) (28.4685, -6.9769) (28.4749, -6.9776) (28.4814, -6.9783) (28.4879, -6.9789) (28.4945, -6.9796) (28.5011, -6.9803) (28.5078, -6.9809) (28.5146, -6.9816) (28.5214, -6.9822) (28.5283, -6.9828) (28.5353, -6.9835) (28.5423, -6.9841) (28.5493, -6.9847) (28.5564, -6.9853) (28.5636, -6.9859) (28.5709, -6.9865) (28.5781, -6.9871) (28.5855, -6.9877) (28.5929, -6.9882) (28.6004, -6.9888) (28.6079, -6.9894) (28.6154, -6.9899) (28.6231, -6.9905) (28.6307, -6.991) (28.6385, -6.9915) (28.6463, -6.9921) (28.6541, -6.9926) (28.662, -6.9931) (28.67, -6.9936) (28.678, -6.994) (28.686, -6.9945) (28.6941, -6.995) (28.7023, -6.9954) (28.7105, -6.9959) (28.7187, -6.9963) (28.727, -6.9968) (28.7354, -6.9972) (28.7438, -6.9976) (28.7523, -6.998) (28.7608, -6.9984) (28.7694, -6.9987) (28.778, -6.9991) (28.7866, -6.9995) (28.7953, -6.9998) (28.8041, -7.0001) (28.8129, -7.0005) (28.8218, -7.0008) (28.8307, -7.0011) (28.8396, -7.0014) (28.8486, -7.0016) (28.8577, -7.0019) (28.8668, -7.0021) (28.8759, -7.0024) (28.8851, -7.0026) (28.8943, -7.0028) (28.9036, -7.003) (28.9129, -7.0032) (28.9223, -7.0034) (28.9317, -7.0036) (28.9412, -7.0037) (28.9507, -7.0038) (28.9602, -7.004) (28.9698, -7.0041) (28.9795, -7.0042) (28.9892, -7.0043) (28.9989, -7.0043) (29.0087, -7.0044) (29.0185, -7.0044) (29.0284, -7.0045) (29.0383, -7.0045) (29.0482, -7.0045) (29.0582, -7.0045) (29.0682, -7.0044) (29.0783, -7.0044) (29.0884, -7.0043) (29.0986, -7.0043) (29.1088, -7.0042) (29.119, -7.0041) (29.1293, -7.004) (29.1396, -7.0038) (29.15, -7.0037) (29.1604, -7.0035) (29.1708, -7.0034) (29.1813, -7.0032) (29.1919, -7.003) (29.2024, -7.0028) (29.213, -7.0025) (29.2237, -7.0023) (29.2344, -7.002) (29.2451, -7.0017) (29.2559, -7.0014) (29.2667, -7.0011) (29.2775, -7.0008) (29.2884, -7.0004) (29.2993, -7.0001) (29.3103, -6.9997) (29.3213, -6.9993) (29.3323, -6.9989) (29.3434, -6.9984) (29.3545, -6.998) (29.3657, -6.9975) (29.3768, -6.997) (29.3881, -6.9965) (29.3993, -6.996) (29.4106, -6.9955) (29.422, -6.995) (29.4333, -6.9944) (29.4447, -6.9938) (29.4562, -6.9932) (29.4677, -6.9926) (29.4792, -6.992) (29.4907, -6.9913) (29.5023, -6.9906) (29.514, -6.99) (29.5256, -6.9892) (29.5373, -6.9885) (29.549, -6.9878) (29.5608, -6.987) (29.5726, -6.9863) (29.5844, -6.9855) (29.5963, -6.9846) (29.6082, -6.9838) (29.6201, -6.983) (29.6321, -6.9821) (29.6441, -6.9812) (29.6562, -6.9803) (29.6682, -6.9794) (29.6803, -6.9784) (29.6925, -6.9775) (29.7047, -6.9765) (29.7169, -6.9755) (29.7291, -6.9745) (29.7414, -6.9735) (29.7537, -6.9724) (29.766, -6.9713) (29.7784, -6.9702) (29.7908, -6.9691) (29.8032, -6.968) (29.8157, -6.9669) (29.8282, -6.9657) (29.8407, -6.9645) (29.8533, -6.9633) (29.8659, -6.9621) (29.8785, -6.9608) (29.8912, -6.9596) (29.9039, -6.9583) (29.9166, -6.957) (29.9293, -6.9556) (29.9421, -6.9543) (29.9549, -6.9529) (29.9678, -6.9516) (29.9806, -6.9501) (29.9935, -6.9487) (30.0065, -6.9473) (30.0194, -6.9458) (30.0324, -6.9443) (30.0455, -6.9428) (30.0585, -6.9413) (30.0716, -6.9398) (30.0847, -6.9382) (30.0979, -6.9366) (30.111, -6.935) (30.1242, -6.9334) (30.1375, -6.9317) (30.1507, -6.9301) (30.164, -6.9284) (30.1773, -6.9267) (30.1907, -6.925) (30.2014, -6.9236) (30.2094, -6.9225) (30.2148, -6.9218) (30.2174, -6.9214) knots 0 0 0 0 0 0 0.00416667 0.00833333 0.0125 0.01666667 0.02083333 0.025 0.02916667 0.03333333 0.0375 0.04166667 0.04583333 0.05 0.05416667 0.05833333 0.0625 0.06666667 0.07083333 0.075 0.07916667 0.08333333 0.0875 0.09166667 0.09583333 0.1 0.10416667 0.10833333 0.1125 0.11666667 0.12083333 0.125 0.12916667 0.13333333 0.1375 0.14166667 0.14583333 0.15 0.15416667 0.15833333 0.1625 0.16666667 0.17083333 0.175 0.17916667 0.18333333 0.1875 0.19166667 0.19583333 0.2 0.20416667 0.20833333 0.2125 0.21666667 0.22083333 0.225 0.22916667 0.23333333 0.2375 0.24166667 0.24583333 0.25 0.25416667 0.25833333 0.2625 0.26666667 0.27083333 0.275 0.27916667 0.28333333 0.2875 0.29166667 0.29583333 0.3 0.30416667 0.30833333 0.3125 0.31666667 0.32083333 0.325 0.32916667 0.33333333 0.3375 0.34166667 0.34583333 0.35 0.35416667 0.35833333 0.3625 0.36666667 0.37083333 0.375 0.37916667 0.38333333 0.3875 0.39166667 0.39583333 0.4 0.40416667 0.40833333 0.4125 0.41666667 0.42083333 0.425 0.42916667 0.43333333 0.4375 0.44166667 0.44583333 0.45 0.45416667 0.45833333 0.4625 0.46666667 0.47083333 0.475 0.47916667 0.48333333 0.4875 0.49166667 0.49583333 0.5 0.50416667 0.50833333 0.5125 0.51666667 0.52083333 0.525 0.52916667 0.53333333 0.5375 0.54166667 0.54583333 0.55 0.55416667 0.55833333 0.5625 0.56666667 0.57083333 0.575 0.57916667 0.58333333 0.5875 0.59166667 0.59583333 0.6 0.60416667 0.60833333 0.6125 0.61666667 0.62083333 0.625 0.62916667 0.63333333 0.6375 0.64166667 0.64583333 0.65 0.65416667 0.65833333 0.6625 0.66666667 0.67083333 0.675 0.67916667 0.68333333 0.6875 0.69166667 0.69583333 0.7 0.70416667 0.70833333 0.7125 0.71666667 0.72083333 0.725 0.72916667 0.73333333 0.7375 0.74166667 0.74583333 0.75 0.75416667 0.75833333 0.7625 0.76666667 0.77083333 0.775 0.77916667 0.78333333 0.7875 0.79166667 0.79583333 0.8 0.80416667 0.80833333 0.8125 0.81666667 0.82083333 0.825 0.82916667 0.83333333 0.8375 0.84166667 0.84583333 0.85 0.85416667 0.85833333 0.8625 0.86666667 0.87083333 0.875 0.87916667 0.88333333 0.8875 0.89166667 0.89583333 0.9 0.90416667 0.90833333 0.9125 0.91666667 0.92083333 0.925 0.92916667 0.93333333 0.9375 0.94166667 0.94583333 0.95 0.95416667 0.95833333 0.9625 0.96666667 0.97083333 0.975 0.97916667 0.98333333 0.9875 0.99166667 0.99583333 1 1 1 1 1 1
  arc A43 (18.6136, 24.7898) -> (17.8246, 25.363) centre (0, 0) ccw
  line L95 (-24.0271, -16.318) -> (-24.0278, -16.3184)
  arc A44 (-25.8803, -12.5209) -> (-25.3417, -13.578) centre (0, 0) ccw
  line L96 (27.918, -6.8665) -> (28.2039, -6.9368)
  line L97 (28.2039, -6.9368) -> (28.2047, -6.937)
  line L98 (27.8945, -8.0948) -> (27.8937, -8.0945)
  line L99 (27.3243, -9.8469) -> (27.3251, -9.8472)
  arc A45 (27.6109, -8.0125) -> (27.918, -6.8665) centre (0, 0) ccw